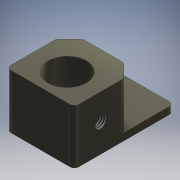
# Autodesk Inventor part: Y End Stop Flag
Saved by Autodesk Inventor 2016 (Build 200138000, 138)
## iProperties
Created: 2017-02-13
Part Number: Y End Stop Flag
Material: PC/ABS Plastic
Document SubType Name: Modeling
Designer: Scott
Density: 0.357273 g/cm^3
Appearance: Gunmetal
Author: Scott
## iProperties of the stored document Y End Stop Flag_3DPrint.ipt
Created: 2017-04-16
Part Number: Y End Stop Flag_3DPrint
Material: Generic
Document SubType Name: Modeling
Designer: Scott
Density: 1 g/cm^3
Appearance: Default
Author: Scott
Autodesk Inventor part; units mm, degrees
ref_plane "YZ Plane" through (0, 0, 0) normal (1, 0, 0) x (0, 1, 0)
ref_plane "XZ Plane" through (0, 0, 0) normal (0, 1, 0) x (-1, 0, 0)
ref_plane "XY Plane" through (0, 0, 0) normal (0, 0, 1) x (1, 0, 0)
sketch "Sketch1" plane through (0, 0, 0) normal (0, 0, 1) x (1, 0, 0)
  circle A0 centre (0, 0) radius 4.25
  line L0 (0, 0) -> (0, 37.2526) construction
  line L1 (0, 0) -> (18.9475, 0) construction
  line L2 (-7.5, 8) -> (7.5, 8)
  line L3 (7.5, 8) -> (7.5, -5.9)
  line L4 (7.5, -5.9) -> (-7.5, -5.9)
  line L5 (-7.5, -5.9) -> (-7.5, 8)
  point P0 (0, 8)
  dimension "d0" = 8.5
  dimension "d1" = 5.9
  dimension "d2" = 15
  dimension "d3" = 8
  constraints: 12 end point, 2 horizontal, 2 parallel, 1 centre point, 1 coincident, 1 midpoint, 1 perpendicular, 1 point on line, 1 vertical
  measures "d0" diameter of A0
  measures "d1" distance from line of L4 L0.start
  measures "d2" distance of L2.start L2.end
  measures "d3" distance from line of L2 L0.start
extrude "Extrusion1" add sketch "Sketch1" along normal blind 12
sketch "Sketch2" plane through (-7.5, 8, 0) normal (0, 1, 0) x (1, 0, 0)
  line L0 (0, 0) -> (15, 0) projected
  line L1 (0, 0) -> (0, -12) projected
  line L2 (15, -12) -> (0, -12) projected
  line L3 (15, 0) -> (15, -12) projected
  line L4 (0, 0) -> (0, -12) projected
  line L5 (0, 0) -> (15, 0)
  line L6 (15, 0) -> (15, -1.6)
  line L7 (15, -1.6) -> (0, -1.6)
  line L8 (0, -1.6) -> (0, 0)
  point P0 (7.5, 0)
  dimension "d6" = 1.6
  constraints: 8 end point, 2 parallel, 1 horizontal, 1 perpendicular, 1 point on line
  measures "d6" distance between parallel lines of L0 L7
extrude "Extrusion2" add sketch "Sketch2" along normal blind 8 contours L0 L3 L7 L1
sketch "Sketch3" plane through (7.5, -5.9, 12) normal (1, 0, 0) x (0, 0, -1)
  line L0 (12, 5.9) -> (-2.61, 5.9) construction
  point P0 (6, 5.9)
  dimension "d9" = 6
  constraints: 2 end point, 1 horizontal, 1 point on line
  measures "d9" distance of L0.start point (6, 5.9)
hole "Hole1" at (7.5, 0, 6) direction (-1, 0, 0) diameter 2.5 end through all
thread "Thread1" size "M3x0.5" class "6H" standard "ANSI Metric M Profile" full length
chamfer "Chamfer1" distance 3 angle 45 2 edges at (7.5, 8, 6.8) (-7.5, 8, 6.8)
fillet "Fillet1" radius 1 4 edges at (-7.5, 16, 0.8) (-4.5, 8, 6.8) (-7.5, 5, 6.8) (-7.5, -5.9, 6)
fillet "Fillet2" radius 1 4 edges at (4.5, 8, 6.8) (7.5, 5, 6.8) (7.5, -5.9, 6) (7.5, 16, 0.8)
body "Solid1"
